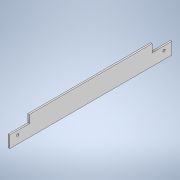
# Autodesk Inventor part: plateHolder
Saved by Autodesk Inventor 2020 (Build 240168000, 168)
## iProperties
Created: 2019-06-19
Part Number: plateHolder
Material: Generic
Document SubType Name: Modeling
Designer: Vivek Muskan
Density: 1 g/cm^3
Appearance: Default
Author: Vivek Muskan
Autodesk Inventor part; units mm, degrees
ref_plane "YZ Plane" through (0, 0, 0) normal (1, 0, 0) x (0, 1, 0)
ref_plane "XZ Plane" through (0, 0, 0) normal (0, 1, 0) x (-1, 0, 0)
ref_plane "XY Plane" through (0, 0, 0) normal (0, 0, 1) x (1, 0, 0)
sketch "Sketch2" plane through (0, 0, 0) normal (1, 0, 0) x (0, 1, 0)
  line L0 (0, 0) -> (-40, 0)
  line L1 (-40, 0) -> (-40, -205)
  line L2 (-40, -205) -> (0, -205)
  line L3 (0, -205) -> (0, 0)
  line L4 (0, 0) -> (0, -5)
  line L5 (0, -5) -> (-5, -5)
  circle A0 centre (-5, -5) radius 1.5
  line L6 (-5, -5) -> (-5, -15)
  circle A1 centre (-5, -15) radius 1.5
  line L7 (0, -102.5) -> (-40, -102.5)
  circle A2 centre (-5, -200) radius 1.5
  circle A3 centre (-5, -190) radius 1.5
  line L8 (-40, 0) -> (-40, -10)
  line L9 (-40, -10) -> (-30, -10)
  line L10 (-30, -10) -> (-20, -10)
  circle A4 centre (-20, -10) radius 1.5
  circle A5 centre (-30, -10) radius 1.5
  circle A6 centre (-20, -195) radius 1.5
  circle A7 centre (-30, -195) radius 1.5
  dimension "d11" = 40
  dimension "d12" = 205
  dimension "d13" = 5
  dimension "d14" = 5
  dimension "d15" = 3
  dimension "d16" = 10
  dimension "d17" = 3
  dimension "d18" = 10
  dimension "d19" = 10
  dimension "d20" = 10
  dimension "d21" = 3
  dimension "d22" = 3
  constraints: 22 end point, 8 centre point, 4 coincident, 4 symmetric about line, 3 perpendicular, 3 point on line, 2 midpoint, 2 parallel, 1 horizontal, 1 vertical, 4 other
  measures "d11" distance of L2.end L1.end
  measures "d12" distance of L1.end L0.end
  measures "d13" distance of L0.start L4.end
  measures "d14" distance of L4.end L5.end
  measures "d15" diameter of A0
  measures "d16" distance of L6.start L6.end
  measures "d17" diameter of A1
  measures "d18" distance of L0.end L8.end
  measures "d19" distance of L8.end L9.end
  measures "d20" distance of L9.end L10.end
  measures "d21" diameter of A4
  measures "d22" diameter of A5
extrude "Extrusion3" add sketch "Sketch2" along normal blind 2
sketch "Sketch3" plane through (2, 0, 0) normal (1, 0, 0) x (0, 0, -1)
  line L0 (205, -40) -> (205, 0) projected
  line L1 (0, 0) -> (205, 0)
  line L2 (205, 0) -> (205, -15)
  line L3 (205, -15) -> (0, -15)
  line L4 (0, -15) -> (0, 0)
  dimension "d25" = 15
  constraints: 8 end point, 2 parallel, 1 horizontal, 1 perpendicular, 1 point on line
  measures "d25" distance of L1.end L2.end
extrude "Extrusion4" cut sketch "Sketch3" against normal blind 2
sketch "Sketch4" plane through (2, 0, 0) normal (1, 0, 0) x (0, 0, -1)
  line L0 (0, -15) -> (0, -40) projected
  line L1 (0, -15) -> (25, -15)
  line L2 (0, -15) -> (205, -15) projected
  line L3 (25, -15) -> (25, -25)
  line L4 (25, -25) -> (0, -25)
  line L5 (205, -40) -> (205, -15) projected
  line L6 (205, -15) -> (180, -15)
  line L7 (180, -15) -> (180, -25)
  line L8 (180, -25) -> (205, -25)
  line L9 (205, -25) -> (205, -15)
  point P0 (0, 0)
  dimension "d28" = 25
  dimension "d29" = 10
  dimension "d30" = 25
  constraints: 14 end point, 3 perpendicular, 2 parallel, 2 point on line, 1 horizontal
  measures "d28" distance of L0.start L1.end
  measures "d29" distance of L1.end L3.end
  measures "d30" distance of L8.end L7.end
extrude "Extrusion5" cut sketch "Sketch4" against normal blind 2
body "Solid2"
